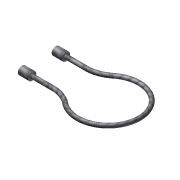
# Autodesk Inventor part: cabo_aco_1
Saved by Autodesk Inventor 2012 SP2 (Build 160219200, 219)
## iProperties
Created: 2015-05-27
Part Number: cabo_aco_1
Material: Default
Document SubType Name: Modeling
Designer: Projeto02
Density: 1 g/cm^3
Author: Projeto02
Autodesk Inventor part; units mm, degrees
ref_plane "YZ Plane" through (0, 0, 0) normal (1, 0, 0) x (0, 1, 0)
ref_plane "XZ Plane" through (0, 0, 0) normal (0, 1, 0) x (-1, 0, 0)
ref_plane "XY Plane" through (0, 0, 0) normal (0, 0, 1) x (1, 0, 0)
sketch "Esboço1" plane through (0, 0, 0) normal (0, 0, 1) x (1, 0, 0)
  arc A0 (19.4794, -3.375) -> (19.4794, 19.875) centre (28.9588, 8.25) ccw
  line L0 (0, 0) -> (10, 0)
  line L1 (0, 16.5) -> (10, 16.5)
  arc A1 (10, 16.5) -> (19.4794, 19.875) centre (10, 31.5) ccw
  arc A2 (19.4794, -3.375) -> (10, 0) centre (10, -15) ccw
  point P0 (16.4314, 16.5)
  point P1 (16.4314, 0)
  dimension "d6" = 16.5
  dimension "d7" = 8.25
  dimension "d8" = 15
  dimension "d9" = 15
  dimension "d10" = 10
  constraints: 8 point on circle, 4 end point, 4 tangent, 3 centre point, 2 point on line, 1 equal radius
  measures "d6" distance between parallel lines of L1 L0
  measures "d7" distance from line of L1 A0.centre
  measures "d8" radius of A0
  measures "d9" radius of A1
  measures "d10" distance of L0.start L0.end
sketch "Esboço2" plane through (0, 0, 0) normal (1, 0, 0) x (0, 1, 0)
  circle A0 centre (0, 0) radius 1
  dimension "d11" = 2
  constraints: 1 centre point, 1 coincident
  measures "d11" diameter of A0
sweep "Varredura1" add profiles "Esboço2" path "Esboço1"
sketch "Esboço3" plane through (0, 0, 0) normal (-1, 0, 0) x (0, 0, 1)
  circle A0 centre (0, 0) radius 1 projected
  circle A1 centre (0, 0) radius 2
  circle A2 centre (0, 16.5) radius 1 projected
  circle A3 centre (0, 16.5) radius 2
  dimension "d13" = 4
  dimension "d14" = 4
  constraints: 2 centre point, 2 coincident
  measures "d13" diameter of A1
  measures "d14" diameter of A3
extrude "Extrusão1" add sketch "Esboço3" along normal blind 5 contours A0 | A1 | A2 | A3
equation "\"d7\" = 0.5 * d6"
equation "\"d13\" = d14"
equation "\"d5\" = 0.5 * d4"
equation "\"d4\" = 16.5"
